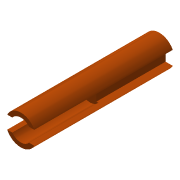
# Autodesk Inventor part: thick rod
Saved by Autodesk Inventor 2016 (Build 200138000, 138)
## iProperties
Created: 2016-07-27
Part Number: thick rod
Material: Polyethylene, High Density
Document SubType Name: Modeling
Designer: dingx
Density: 0.952 g/cm^3
Appearance: Smooth - Light Orange
Author: dingx
Autodesk Inventor part; units mm, degrees
ref_plane "YZ Plane" through (0, 0, 0) normal (1, 0, 0) x (0, 1, 0)
ref_plane "XZ Plane" through (0, 0, 0) normal (0, 1, 0) x (-1, 0, 0)
ref_plane "XY Plane" through (0, 0, 0) normal (0, 0, 1) x (1, 0, 0)
sketch "Sketch1" plane through (0, 0, 0) normal (0, 0, 1) x (1, 0, 0)
  arc A0 (-1.5748, -2.3876) -> (-1.5748, 2.3876) centre (-1.5748, 0) ccw
  line L0 (-1.5748, 2.3876) -> (-5.0101, 2.3876)
  line L1 (-1.5748, -2.3876) -> (-5.0101, -2.3876)
  line L2 (2.286, -2.54) -> (2.286, 2.54)
  line L3 (2.286, 2.54) -> (4.9346, 2.54)
  line L4 (2.286, -2.54) -> (4.9346, -2.54)
  arc A1 (-5.0101, -2.3876) -> (4.9346, -2.54) centre (0, 0) ccw
  arc A2 (4.9346, 2.54) -> (-5.0101, 2.3876) centre (0, 0) ccw
  point P0 (2.286, 0)
  dimension "d1" = 4.7752
  dimension "d2" = 1.5748
  dimension "d3" = 5.08
  dimension "d4" = 2.286
  dimension "d10" = 5.5499
  dimension "d11" = 5.5499
  dimension "d12" = 0.1524
  constraints: 10 end point, 6 point on circle, 3 centre point, 2 horizontal, 2 parallel, 2 tangent, 1 coincident, 1 horizontal alignment, 1 midpoint, 1 vertical
  measures "d1" diameter of A0
  measures "d2" distance of point (0, 0) A0.centre
  measures "d3" distance of L2.start L2.end
  measures "d4" distance of point (2.286, 0) point (0, 0)
  measures "d10" radius of A1
  measures "d11" radius of A2
  measures "d12" distance between parallel lines of L0 L3
extrude "Extrusion1" add sketch "Sketch1" along normal blind 50.8
sketch "Sketch2" plane through (0, 0, 50.8) normal (0, 0, 1) x (1, 0, 0)
  circle A0 centre (0, 0) radius 3.9624
  dimension "d7" = 7.9248
  constraints: 1 centre point, 1 coincident
  measures "d7" diameter of A0
extrude "Extrusion2" cut sketch "Sketch2" against normal blind 25.4
body "Solid1"
